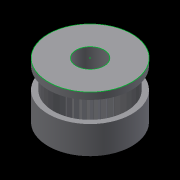
# Autodesk Inventor part: XY gear
Saved by Autodesk Inventor 2014 (Build 180170000, 170)
## iProperties
Created: 2014-11-07
Part Number: XY gear
Material: Generic
Document SubType Name: Modeling
Designer: Scott
Density: 1 g/cm^3
Appearance: Default
Author: Scott
Autodesk Inventor part; units mm, degrees
ref_plane "YZ Plane" through (0, 0, 0) normal (1, 0, 0) x (0, 1, 0)
ref_plane "XZ Plane" through (0, 0, 0) normal (0, 1, 0) x (-1, 0, 0)
ref_plane "XY Plane" through (0, 0, 0) normal (0, 0, 1) x (1, 0, 0)
sketch "Sketch1" plane through (0, 0, 0) normal (0, 1, 0) x (-1, 0, 0)
  circle A0 centre (0, 0) radius 2.54
  circle A1 centre (0, 0) radius 5.969
  dimension "d0" = 5.08
  constraints: 2 centre point, 2 coincident
  measures "d0" diameter of A0
extrude "Extrusion1" add sketch "Sketch1" along normal blind 10.16
sketch "Sketch2" plane through (0, 10.16, 0) normal (0, 1, 0) x (1, 0, 0)
  circle A0 centre (0, 0) radius 2.54 projected
  circle A1 centre (0, 0) radius 5.969 projected
  line L0 (2.54, 0) -> (6.731, 0)
  circle A2 centre (0, 0) radius 6.731
  dimension "d4" = 4.191
  constraints: 2 end point, 2 horizontal alignment, 1 coincident, 1 horizontal, 3 other
  measures "d4" distance of L0.start L0.end
extrude "Extrusion2" add sketch "Sketch2" against normal blind 1.27 contours A2
sketch "Sketch3" plane through (0, 0, 0) normal (0, -1, 0) x (1, 0, 0)
  circle A0 centre (0, 0) radius 5.969 projected
  circle A1 centre (0, 0) radius 6.6711
  constraints: 1 centre point, 1 coincident
extrude "Extrusion3" add sketch "Sketch3" against normal blind 3.81
sketch "Sketch4" plane through (0, 3.81, 0) normal (0, 1, 0) x (1, 0, 0)
  circle A0 centre (0, 0) radius 5.969 projected
  circle A1 centre (0, 0) radius 6.6711 projected
  line L0 (5.969, 0.0012) -> (5.3134, 0.0012)
  line L1 (5.3134, 0.0012) -> (5.3134, -0.4433)
  line L2 (5.9525, -0.4433) -> (6.6711, 0.0012)
  line L3 (6.6711, 0.0012) -> (5.9525, 0.4433)
  arc A2 (5.9525, -0.4433) -> (5.9525, 0.4433) centre (0, 0) ccw
  line L4 (5.9486, 0.4934) -> (6.5888, 1.0448)
  line L5 (6.5888, 1.0448) -> (5.8099, 1.369)
  arc A3 (5.9486, 0.4934) -> (5.8099, 1.369) centre (0, 0) ccw
  line L6 (5.7982, 1.4179) -> (6.3443, 2.0627)
  line L7 (6.3443, 2.0627) -> (5.5242, 2.261)
  arc A4 (5.7982, 1.4179) -> (5.5242, 2.261) centre (0, 0) ccw
  line L8 (5.505, 2.3074) -> (5.9435, 3.0297)
  line L9 (5.9435, 3.0297) -> (5.1025, 3.0973)
  arc A5 (5.505, 2.3074) -> (5.1025, 3.0973) centre (0, 0) ccw
  line L10 (5.0762, 3.1402) -> (5.3963, 3.9222)
  line L11 (5.3963, 3.9222) -> (4.5551, 3.8574)
  arc A6 (5.0762, 3.1402) -> (4.5551, 3.8574) centre (0, 0) ccw
  line L12 (4.5225, 3.8956) -> (4.7163, 4.7181)
  line L13 (4.7163, 4.7181) -> (3.8956, 4.5225)
  arc A7 (4.5225, 3.8956) -> (3.8956, 4.5225) centre (0, 0) ccw
  line L14 (3.8574, 4.5551) -> (3.9202, 5.3978)
  line L15 (3.9202, 5.3978) -> (3.1402, 5.0762)
  arc A8 (3.8574, 4.5551) -> (3.1402, 5.0762) centre (0, 0) ccw
  line L16 (3.0973, 5.1025) -> (3.0275, 5.9446)
  line L17 (3.0275, 5.9446) -> (2.3074, 5.505)
  arc A9 (3.0973, 5.1025) -> (2.3074, 5.505) centre (0, 0) ccw
  line L18 (2.261, 5.5242) -> (2.0603, 6.345)
  line L19 (2.0603, 6.345) -> (1.4179, 5.7982)
  arc A10 (2.261, 5.5242) -> (1.4179, 5.7982) centre (0, 0) ccw
  line L20 (1.369, 5.8099) -> (1.0424, 6.5892)
  line L21 (1.0424, 6.5892) -> (0.4934, 5.9486)
  arc A11 (1.369, 5.8099) -> (0.4934, 5.9486) centre (0, 0) ccw
  line L22 (0.4433, 5.9525) -> (-0.0012, 6.6711)
  line L23 (-0.0012, 6.6711) -> (-0.4433, 5.9525)
  arc A12 (0.4433, 5.9525) -> (-0.4433, 5.9525) centre (0, 0) ccw
  line L24 (-0.4934, 5.9486) -> (-1.0448, 6.5888)
  line L25 (-1.0448, 6.5888) -> (-1.369, 5.8099)
  arc A13 (-0.4934, 5.9486) -> (-1.369, 5.8099) centre (0, 0) ccw
  line L26 (-1.4179, 5.7982) -> (-2.0627, 6.3443)
  line L27 (-2.0627, 6.3443) -> (-2.261, 5.5242)
  arc A14 (-1.4179, 5.7982) -> (-2.261, 5.5242) centre (0, 0) ccw
  line L28 (-2.3074, 5.505) -> (-3.0297, 5.9435)
  line L29 (-3.0297, 5.9435) -> (-3.0973, 5.1025)
  arc A15 (-2.3074, 5.505) -> (-3.0973, 5.1025) centre (0, 0) ccw
  line L30 (-3.1402, 5.0762) -> (-3.9222, 5.3963)
  line L31 (-3.9222, 5.3963) -> (-3.8574, 4.5551)
  arc A16 (-3.1402, 5.0762) -> (-3.8574, 4.5551) centre (0, 0) ccw
  line L32 (-3.8956, 4.5225) -> (-4.7181, 4.7163)
  line L33 (-4.7181, 4.7163) -> (-4.5225, 3.8956)
  arc A17 (-3.8956, 4.5225) -> (-4.5225, 3.8956) centre (0, 0) ccw
  line L34 (-4.5551, 3.8574) -> (-5.3978, 3.9202)
  line L35 (-5.3978, 3.9202) -> (-5.0762, 3.1402)
  arc A18 (-4.5551, 3.8574) -> (-5.0762, 3.1402) centre (0, 0) ccw
  line L36 (-5.1025, 3.0973) -> (-5.9446, 3.0275)
  line L37 (-5.9446, 3.0275) -> (-5.505, 2.3074)
  arc A19 (-5.1025, 3.0973) -> (-5.505, 2.3074) centre (0, 0) ccw
  line L38 (-5.5242, 2.261) -> (-6.345, 2.0603)
  line L39 (-6.345, 2.0603) -> (-5.7982, 1.4179)
  arc A20 (-5.5242, 2.261) -> (-5.7982, 1.4179) centre (0, 0) ccw
  line L40 (-5.8099, 1.369) -> (-6.5892, 1.0424)
  line L41 (-6.5892, 1.0424) -> (-5.9486, 0.4934)
  arc A21 (-5.8099, 1.369) -> (-5.9486, 0.4934) centre (0, 0) ccw
  line L42 (-5.9525, 0.4433) -> (-6.6711, -0.0012)
  line L43 (-6.6711, -0.0012) -> (-5.9525, -0.4433)
  arc A22 (-5.9525, 0.4433) -> (-5.9525, -0.4433) centre (0, 0) ccw
  line L44 (-5.9486, -0.4934) -> (-6.5888, -1.0448)
  line L45 (-6.5888, -1.0448) -> (-5.8099, -1.369)
  arc A23 (-5.9486, -0.4934) -> (-5.8099, -1.369) centre (0, 0) ccw
  line L46 (-5.7982, -1.4179) -> (-6.3443, -2.0627)
  line L47 (-6.3443, -2.0627) -> (-5.5242, -2.261)
  arc A24 (-5.7982, -1.4179) -> (-5.5242, -2.261) centre (0, 0) ccw
  line L48 (-5.505, -2.3074) -> (-5.9435, -3.0297)
  line L49 (-5.9435, -3.0297) -> (-5.1025, -3.0973)
  arc A25 (-5.505, -2.3074) -> (-5.1025, -3.0973) centre (0, 0) ccw
  line L50 (-5.0762, -3.1402) -> (-5.3963, -3.9222)
  line L51 (-5.3963, -3.9222) -> (-4.5551, -3.8574)
  arc A26 (-5.0762, -3.1402) -> (-4.5551, -3.8574) centre (0, 0) ccw
  line L52 (-4.5225, -3.8956) -> (-4.7163, -4.7181)
  line L53 (-4.7163, -4.7181) -> (-3.8956, -4.5225)
  arc A27 (-4.5225, -3.8956) -> (-3.8956, -4.5225) centre (0, 0) ccw
  line L54 (-3.8574, -4.5551) -> (-3.9202, -5.3978)
  line L55 (-3.9202, -5.3978) -> (-3.1402, -5.0762)
  arc A28 (-3.8574, -4.5551) -> (-3.1402, -5.0762) centre (0, 0) ccw
  line L56 (-3.0973, -5.1025) -> (-3.0275, -5.9446)
  line L57 (-3.0275, -5.9446) -> (-2.3074, -5.505)
  arc A29 (-3.0973, -5.1025) -> (-2.3074, -5.505) centre (0, 0) ccw
  line L58 (-2.261, -5.5242) -> (-2.0603, -6.345)
  line L59 (-2.0603, -6.345) -> (-1.4179, -5.7982)
  arc A30 (-2.261, -5.5242) -> (-1.4179, -5.7982) centre (0, 0) ccw
  line L60 (-1.369, -5.8099) -> (-1.0424, -6.5892)
  line L61 (-1.0424, -6.5892) -> (-0.4934, -5.9486)
  arc A31 (-1.369, -5.8099) -> (-0.4934, -5.9486) centre (0, 0) ccw
  line L62 (-0.4433, -5.9525) -> (0.0012, -6.6711)
  line L63 (0.0012, -6.6711) -> (0.4433, -5.9525)
  arc A32 (-0.4433, -5.9525) -> (0.4433, -5.9525) centre (0, 0) ccw
  line L64 (0.4934, -5.9486) -> (1.0448, -6.5888)
  line L65 (1.0448, -6.5888) -> (1.369, -5.8099)
  arc A33 (0.4934, -5.9486) -> (1.369, -5.8099) centre (0, 0) ccw
  line L66 (1.4179, -5.7982) -> (2.0627, -6.3443)
  line L67 (2.0627, -6.3443) -> (2.261, -5.5242)
  arc A34 (1.4179, -5.7982) -> (2.261, -5.5242) centre (0, 0) ccw
  line L68 (2.3074, -5.505) -> (3.0297, -5.9435)
  line L69 (3.0297, -5.9435) -> (3.0973, -5.1025)
  arc A35 (2.3074, -5.505) -> (3.0973, -5.1025) centre (0, 0) ccw
  line L70 (3.1402, -5.0762) -> (3.9222, -5.3963)
  line L71 (3.9222, -5.3963) -> (3.8574, -4.5551)
  arc A36 (3.1402, -5.0762) -> (3.8574, -4.5551) centre (0, 0) ccw
  line L72 (3.8956, -4.5225) -> (4.7181, -4.7163)
  line L73 (4.7181, -4.7163) -> (4.5225, -3.8956)
  arc A37 (3.8956, -4.5225) -> (4.5225, -3.8956) centre (0, 0) ccw
  line L74 (4.5551, -3.8574) -> (5.3978, -3.9202)
  line L75 (5.3978, -3.9202) -> (5.0762, -3.1402)
  arc A38 (4.5551, -3.8574) -> (5.0762, -3.1402) centre (0, 0) ccw
  line L76 (5.1025, -3.0973) -> (5.9446, -3.0275)
  line L77 (5.9446, -3.0275) -> (5.505, -2.3074)
  arc A39 (5.1025, -3.0973) -> (5.505, -2.3074) centre (0, 0) ccw
  line L78 (5.5242, -2.261) -> (6.345, -2.0603)
  line L79 (6.345, -2.0603) -> (5.7982, -1.4179)
  arc A40 (5.5242, -2.261) -> (5.7982, -1.4179) centre (0, 0) ccw
  line L80 (5.8099, -1.369) -> (6.5892, -1.0424)
  line L81 (6.5892, -1.0424) -> (5.9486, -0.4934)
  arc A41 (5.8099, -1.369) -> (5.9486, -0.4934) centre (0, 0) ccw
  point P0 (5.8953, 0.935)
  point P1 (5.6765, 1.8457)
  point P2 (5.3179, 2.711)
  point P3 (4.8283, 3.5095)
  point P4 (4.2199, 4.2216)
  point P5 (3.5075, 4.8297)
  point P6 (2.7088, 5.319)
  point P7 (1.8434, 5.6772)
  point P8 (0.9325, 5.8957)
  point P9 (-0.0012, 5.969)
  point P10 (-0.935, 5.8953)
  point P11 (-1.8457, 5.6765)
  point P12 (-2.711, 5.3179)
  point P13 (-3.5095, 4.8283)
  point P14 (-4.2216, 4.2199)
  point P15 (-4.8297, 3.5075)
  point P16 (-5.319, 2.7088)
  point P17 (-5.6772, 1.8434)
  point P18 (-5.8957, 0.9325)
  point P19 (-5.969, -0.0012)
  point P20 (-5.8953, -0.935)
  point P21 (-5.6765, -1.8457)
  point P22 (-5.3179, -2.711)
  point P23 (-4.8283, -3.5095)
  point P24 (-4.2199, -4.2216)
  point P25 (-3.5075, -4.8297)
  point P26 (-2.7088, -5.319)
  point P27 (-1.8434, -5.6772)
  point P28 (-0.9325, -5.8957)
  point P29 (0.0012, -5.969)
  point P30 (0.935, -5.8953)
  point P31 (1.8457, -5.6765)
  point P32 (2.711, -5.3179)
  point P33 (3.5095, -4.8283)
  point P34 (4.2216, -4.2199)
  point P35 (4.8297, -3.5075)
  point P36 (5.319, -2.7088)
  point P37 (5.6772, -1.8434)
  point P38 (5.8957, -0.9325)
  dimension "d9" = 0.4445
  dimension "d12" = 360
  constraints: 164 end point, 123 point on circle, 40 centre point, 1 perpendicular, 323 other
  measures "d9" distance of L0.end L1.end
extrude "Extrusion4" add sketch "Sketch4" along normal blind 5.08 contours A0 L3 L2 | A0 L5 L4 | L81 L80 A0 | A0 L7 L6 | L78 A0 L79 | L8 A0 L9 | L76 A0 L77 | L10 A0 L11 | L74 A0 L75 | L12 A0 L13 | L72 A0 L73 | L14 A0 L15 | L70 A0 L71 | L16 A0 L17 | L68 A0 L69 | L18 A0 L19 | L66 A0 L67 | L20 A0 L21 | L64 A0 L65 | L22 A0 L23 | L62 A0 L63 | L24 A0 L25 | L60 A0 L61 | L26 A0 L27 | L58 A0 L59 | L28 A0 L29 | L56 A0 L57 | L30 A0 L31 | L54 A0 L55 | L32 A0 L33 | L52 A0 L53 | L34 A0 L35 | L50 A0 L51 | L36 A0 L37 | L48 A0 L49 | L38 A0 L39 | L46 A0 L47 | L40 A0 L41 | L44 A0 L45 | L42 A0 L43
sketch "Sketch5" plane through (0, 0, 0) normal (0, -1, 0) x (1, 0, 0)
  circle A0 centre (0, 0) radius 6.6711 projected
  circle A1 centre (0, 0) radius 2.54 projected
  circle A2 centre (0, 0) radius 7.62
  dimension "d16" = 15.24
  constraints: 1 centre point, 1 coincident
  measures "d16" diameter of A2
extrude "Extrusion5" add sketch "Sketch5" against normal blind 5.08 contours A2
sketch "Sketch6" plane through (0, 10.16, 0) normal (0, 1, 0) x (1, 0, 0)
  circle A0 centre (0, 0) radius 6.731 projected
  circle A1 centre (0, 0) radius 2.54 projected
  circle A2 centre (0, 0) radius 7.62
  dimension "d19" = 15.24
  constraints: 1 centre point, 1 coincident
  measures "d19" diameter of A2
extrude "Extrusion6" add sketch "Sketch6" against normal blind 1.27 contours A2
sketch "Sketch7" plane through (0, 10.16, 0) normal (0, 1, 0) x (1, 0, 0)
  circle A0 centre (0, 0) radius 7.62 projected
  circle A1 centre (0, 0) radius 2.54 projected
body "Solid1"
